Autodesk Inventor part; units mm, degrees
(part 2 of 2)
equation "\"d26\" = allenKeyHole2_5mm"
equation "\"d27\" = allenKeyHole2_0mm"
equation "\"d28\" = allenKeyHold1_5mm"
equation "\"d34\" = depthOfLetters"
equation "\"innerDiameter\" = 31.75"
equation "\"edgeRadius\" = 4.699"
equation "\"allenKey3_0mm\" = 3"
equation "\"allenKeyClearance\" = 0.5"
equation "\"allenKeyHole3_0mm\" = allenKey3_0mm + allenKeyClearance"
equation "\"screwRadius\" = 0.5 * innerDiameter + 0.5 * edgeRadius"
equation "\"allenKey4_0mm\" = 4"
equation "\"allenKey3_5mm\" = 3.5"
equation "\"allenKey2_5mm\" = 2.5"
equation "\"alleyKey2_0mm\" = 2"
equation "\"allenKey1_5mm\" = 1.5"
equation "\"allenKeyHole4_0mm\" = allenKey4_0mm + allenKeyClearance"
equation "\"allenKeyHole2_5mm\" = allenKey2_5mm + allenKeyClearance"
equation "\"allenKeyHole2_0mm\" = alleyKey2_0mm + allenKeyClearance"
equation "\"allenKeyHole3_5mm\" = allenKey3_5mm + allenKeyClearance"
equation "\"allenKeyHold1_5mm\" = allenKey1_5mm + allenKeyClearance"
equation "\"depthWiderTopUnit\" = 9.525"
equation "\"depthLowerUnit\" = 9.525"
equation "\"depthOfLetters\" = 3.175"
equation "\"outerDiameter\" = 41.148"
body "Solid1"
